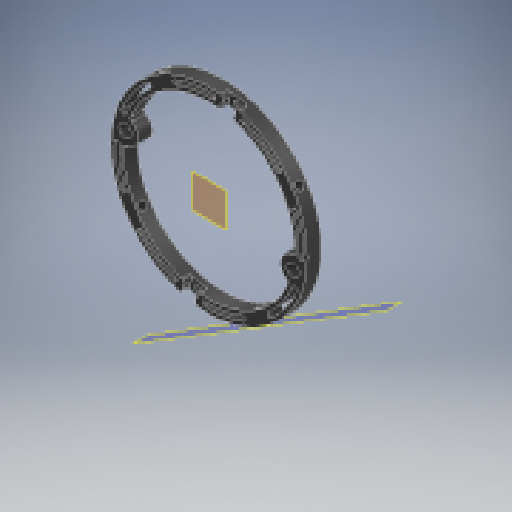
# Autodesk Inventor part: 3DprintRadial
Saved by Autodesk Inventor 2027 (Build 310192060, 192F)
## iProperties
Created: 2026-06-26
Part Number: 3DprintRadial
Material: ABS Plastic
Document SubType Name: Modeling
Designer: opore
Density: 1.06 g/cm^3
Appearance: Default
Author: opore
Autodesk Inventor part; units mm, degrees
ref_plane "YZ Plane" through (0, 0, 0) normal (1, 0, 0) x (0, 1, 0)
ref_plane "XZ Plane" through (0, 0, 0) normal (0, 1, 0) x (-1, 0, 0)
ref_plane "XY Plane" through (0, 0, 0) normal (0, 0, 1) x (1, 0, 0)
sketch "Sketch1" plane through (0, 0, 0) normal (0, 0, 1) x (1, 0, 0)
  circle A0 centre (0, 0) radius 63.2 projected
  circle A1 centre (0, 0) radius 63.2
  circle A2 centre (0, 0) radius 55
  point P0 (0, 0)
  dimension "d0" = 110
  constraints: 2 centre point, 2 coincident, 1 concentric
  measures "d0" diameter of A2
extrude "Extrusion1" add sketch "Sketch1" along normal blind 9
sketch "Sketch2" plane through (0, 0, 9) normal (0, 0, 1) x (1, 0, 0)
  circle A0 centre (53.7689, -11.7651) radius 4.05
  circle A1 centre (-53.7686, 11.7651) radius 4.05
  circle A2 centre (53.7689, -11.7651) radius 8
  circle A3 centre (-53.7686, 11.7651) radius 8
  circle A4 centre (0, 0) radius 63.2 projected
  circle A5 centre (0, 0) radius 55 projected
  point P0 (0, 0)
  point P1 (-54.448, 7.7725)
  point P2 (-54.8657, 3.8406)
  point P3 (-51.4561, 19.4235)
  point P4 (-52.7185, 15.6766)
  point P5 (51.4561, -19.4235)
  point P6 (52.7186, -15.6766)
  point P7 (54.448, -7.7725)
  point P8 (54.8657, -3.8407)
  dimension "d3" = 8.1
  dimension "d4" = 8.1
  dimension "d17" = 16
  dimension "d18" = 16
  constraints: 4 centre point, 2 coincident
  measures "d3" diameter of A0
  measures "d4" diameter of A1
  measures "d17" diameter of A2
  measures "d18" diameter of A3
extrude "Extrusion2" add sketch "Sketch2" against normal blind 9 contours A0 A5 A2 | A5 A1 A3 picked at (53.3566, -6.0588) picked at (-50.6637, 16.5289)
sketch "Sketch3" plane through (0, 0, 9) normal (0, 0, 1) x (1, 0, 0)
  circle A0 centre (53.7689, -11.7651) radius 4.05 projected
  arc A1 (-54.448, 7.7725) -> (-52.7185, 15.6766) centre (-53.7686, 11.7651) ccw projected
  circle A2 centre (-53.7686, 11.7651) radius 4.05 projected
  point P0 (0, 0)
extrude "Extrusion3" cut sketch "Sketch3" against normal blind 9
fillet "Fillet1" radius 2 4 edges at (-51.4561, 19.4235, 4.5) (-54.8657, 3.8406, 4.5) (54.8657, -3.8407, 4.5) (51.4561, -19.4235, 4.5)
ref_plane "Work Plane2" through (33.0646, -53.8607, 0) normal (0.5232, -0.8522, 0) x (0.8522, 0.5232, 0)
ref_plane "Work Plane1" through (27.0345, -7.7211, -32) normal (0.5232, -0.8522, 0) x (0.8522, 0.5232, 0)
sketch "Sketch4" plane through (33.0646, -53.8607, 0) normal (0.5232, -0.8522, 0) x (0.8522, 0.5232, 0)
  line L0 (63.2, 9) -> (-63.2, 9) projected
  line L1 (63.2, 0) -> (-63.2, 0) projected
  line L2 (63.2, 9) -> (-63.2, 9)
  line L3 (0, 0) -> (0, 13.0058)
  line L4 (0, 9) -> (0, 4.5)
  circle A0 centre (0, 4.5) radius 2.6
  dimension "d10" = 4.5
  dimension "d11" = 5.2
  constraints: 6 end point, 2 point on line, 1 centre point, 1 coincident, 1 horizontal, 1 midpoint, 1 vertical
  measures "d10" distance of L4.start L4.end
  measures "d11" diameter of A0
extrude "Extrusion4" cut sketch "Sketch4" against normal blind 9
pattern_circular "Circular Pattern1" count 4 over 360 about axis through (0, 0, 0) along (0, 0, 1) of "Extrusion4"
sketch "Sketch5" plane through (0, 0, 9) normal (0, 0, 1) x (1, 0, 0)
  circle A0 centre (-53.7686, 11.7651) radius 4.05 projected
  circle A1 centre (0, 0) radius 63.2 projected
  arc A2 (54.9684, -1.8649) -> (-50.7242, 21.2617) centre (0, 0) ccw projected
  arc A3 (53.1294, -3.7907) -> (54.9684, -1.8649) centre (52.9695, -1.7971) ccw projected
  arc A4 (53.1294, -3.7907) -> (49.8575, -18.7438) centre (53.7689, -11.7651) ccw projected
  arc A5 (50.7242, -21.2616) -> (49.8575, -18.7438) centre (48.8797, -20.4884) ccw projected
  arc A6 (-54.9684, 1.8648) -> (50.7242, -21.2616) centre (0, 0) ccw projected
  arc A7 (-53.1293, 3.7906) -> (-54.9684, 1.8648) centre (-52.9695, 1.797) ccw projected
  arc A8 (-53.1293, 3.7906) -> (-49.8574, 18.7438) centre (-53.7686, 11.7651) ccw projected
  arc A9 (-50.7242, 21.2617) -> (-49.8574, 18.7438) centre (-48.8797, 20.4885) ccw projected
  circle A10 centre (53.7689, -11.7651) radius 4.05 projected
  line L0 (53.7689, -11.7651) -> (-53.7686, 11.7651)
  line L1 (0, 0) -> (-14.2575, -65.1597)
  circle A11 centre (0, 0) radius 59.1
  circle A12 centre (-12.6327, -57.7341) radius 2
  line L2 (-14.2575, -65.1597) -> (17.2486, 78.8294)
  circle A13 centre (12.6327, 57.7341) radius 2
  point P0 (0, 0)
  dimension "d19" = 90
  dimension "d20" = 118.2
  dimension "d21" = 4
  dimension "d22" = 4
  constraints: 6 end point, 3 centre point, 2 point on circle, 2 point on line, 1 coincident
  measures "d19" angle of L1 L0
  measures "d20" diameter of A11
  measures "d21" diameter of A12
  measures "d22" diameter of A13
extrude "Extrusion5" cut sketch "Sketch5" against normal blind 9 contours A12 A11 L1 | L1 A11 A12 | A13 A11 L2 | L2 A11 A13 | A11 A12 L1 | L1 A12 A11 | L2 A13 A11 | A11 A13 L2
ref_plane "Work Plane4" through (0, 0, 9) normal (0, 0, 1) x (1, 0, 0)
sketch "Sketch6" plane through (0, 0, 9) normal (0, 0, 1) x (1, 0, 0)
  line L0 (0, 0) -> (-76.3563, -46.8744)
  line L1 (-52.4548, -35.2524) -> (-45.4598, -30.9582) projected
  line L2 (0, 0) -> (54.2047, -88.297)
  arc A0 (36.0525, -58.7279) -> (25.5891, -41.6834) centre (30.8208, -50.2057) ccw
  circle A1 centre (-12.6327, -57.7341) radius 2 projected
  arc A2 (-2.718, -59.0375) -> (21.972, -54.8638) centre (0, 0) ccw
  arc A3 (-14.579, -57.2736) -> (-10.672, -58.1285) centre (0, 0) ccw
  arc A4 (30.9196, -50.3666) -> (-48.9575, -33.1054) centre (0, 0) ccw
  arc A5 (-44.4326, -38.9687) -> (-22.1858, -54.7778) centre (0, 0) ccw
  arc A6 (-2.787, -60.5359) -> (22.5297, -56.2563) centre (0, 0) ccw
  arc A7 (-2.6491, -57.5391) -> (21.4143, -53.4714) centre (0, 0) ccw
  arc A8 (-45.5603, -39.9577) -> (-22.7489, -56.168) centre (0, 0) ccw
  arc A9 (-43.3048, -37.9796) -> (-21.6227, -53.3875) centre (0, 0) ccw
  circle A10 centre (-22.1858, -54.7778) radius 1.5
  circle A11 centre (-44.4326, -38.9687) radius 1.5
  circle A12 centre (21.972, -54.8638) radius 1.5011
  circle A13 centre (-2.718, -59.0375) radius 1.5
  point P0 (-21.6227, -53.3875)
  point P1 (22.4761, -56.2778)
  point P2 (21.3621, -53.4922)
  point P3 (-2.6491, -57.5391)
  dimension "d28" = 20
  dimension "d31" = 1.5
  dimension "d32" = 1.5
  dimension "d33" = 1.5
  dimension "d34" = 1.5
  constraints: 21 point on circle, 10 centre point, 5 coincident, 5 point on line, 4 end point, 1 parallel, 9 other
  measures "d28" diameter of A0
  measures "d31" radial gap between concentric circles of A2 A6
  measures "d32" radial gap between concentric circles of A2 A7
  measures "d33" radial gap between concentric circles of A5 A8
  measures "d34" radial gap between concentric circles of A5 A9
extrude "Extrusion6" cut sketch "Sketch6" against normal blind 9 contours A13 A7 A12 A2 | A2 A12 A6 A13 | A13 | A12 | A11 A9 A10 A5 | A5 A10 A8 A11 | A11 | A10
ref_plane "Work Plane3" through (0, 0, 9) normal (0, 0, 1) x (1, 0, 0)
sketch "Sketch8" plane through (0, 0, 9) normal (0, 0, 1) x (1, 0, 0)
  circle A0 centre (-12.6327, -57.7341) radius 2 projected
  circle A1 centre (-12.6327, -57.7341) radius 4.5
  circle A2 centre (12.6327, 57.7341) radius 2.1025 projected
  circle A3 centre (12.6327, 57.7341) radius 4.5
  point P0 (0, 0)
  dimension "d50" = 9
  dimension "d51" = 9
  constraints: 2 centre point, 2 coincident
  measures "d50" diameter of A1
  measures "d51" diameter of A3
extrude "Extrusion7" cut sketch "Sketch8" against normal blind 5 contours A0 | A1 | A2 | A3
fillet "Fillet2" radius 2 4 edges at (-11.6295, -62.1208, 6.5) (-15.3763, -61.301, 6.5) (-13.4978, -53.318, 6.5) (-10.0025, -54.0828, 6.5)
fillet "Fillet3" radius 2 4 edges at (10.0025, 54.0828, 6.5) (13.4978, 53.318, 6.5) (11.6295, 62.1208, 6.5) (15.3763, 61.301, 6.5)
pattern_circular "Circular Pattern3" count 4 over 360 about axis through (0, 0, -10) along (0, 0, 1) of "Extrusion6"
body "Solid1"
